rtholderjoiner (Autodesk Fusion 360 design; units mm, degrees)
Autodesk Fusion 360 part; units mm, degrees
sketch "Sketch1" plane through (0, 0, 0) normal (0, 1, 0) x (1, 0, 0)
  line L0 (-41.6403, -0.018) -> (25.1836, -0.018)
  line L1 (-8.2283, -0.018) -> (-13.2283, -0.018)
  line L2 (-13.2283, -0.018) -> (-13.2283, -5.018)
  line L3 (-13.2283, -5.018) -> (-8.2283, -5.018)
  line L4 (-8.2283, -5.018) -> (-8.2283, -0.018)
  line L5 (6.3716, -0.018) -> (14.3716, -0.018)
  line L6 (14.3716, -0.018) -> (14.3716, -8.018)
  line L7 (14.3716, -8.018) -> (6.3716, -8.018)
  line L8 (6.3716, -8.018) -> (6.3716, -0.018)
  dimension "d1" = 5
  dimension "d2" = 5
  dimension "d3" = 8
  dimension "d4" = 8
  constraint horizontal L0
  constraint horizontal L1
  constraint vertical L2
  constraint horizontal L3
  constraint vertical L4
  constraint midpoint L0 L1.start
  constraint horizontal L5
  constraint vertical L6
  constraint horizontal L7
  constraint vertical L8
  constraint coincident L0 L5.start
  measures "d1" distance of L1.start L1.end
  measures "d2" distance of L1.start L3.end
  measures "d3" distance of L5.start L5.end
  measures "d4" distance of L5.start L7.end
extrude "Extrude1" add sketch "Sketch1" along normal blind 93.6 contours L0 L1 L2 L3 L4 makes body 1
extrude "Extrude2" add sketch "Sketch1" along normal blind 93.6 separate body contours L0 L5 L6 L7 L8 makes body 2
